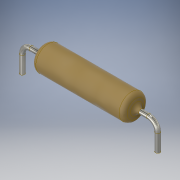
# Autodesk Inventor part: Resistor_TH-15mm
Saved by Autodesk Inventor 2018 (Build 220112000, 112)
## iProperties
Created: 2018-07-06
Part Number: Resistor_TH-15mm
Material: Copper
Document SubType Name: Modeling
Designer: Bradley
Density: 8.94 g/cm^3
Appearance: Textured - Dark Gold
Mass: 1.31337 g
Surface Area: 1.83215 cm^2
Volume: 0.14691 cm^3
Author: Bradley
Autodesk Inventor part; units mm, degrees
ref_plane "YZ Plane" through (0, 0, 0) normal (1, 0, 0) x (0, 1, 0)
ref_plane "XZ Plane" through (0, 0, 0) normal (0, 1, 0) x (-1, 0, 0)
ref_plane "XY Plane" through (0, 0, 0) normal (0, 0, 1) x (1, 0, 0)
sketch "Sketch1" plane through (0, 0, 0) normal (0, 0, 1) x (1, 0, 0)
  line L0 (-5.6474, 0) -> (5.6474, 0)
  line L1 (5.6474, 0) -> (5.6474, 0.254)
  arc A0 (5.155, 0.6672) -> (5.6474, 0.254) centre (5.6474, 0.754) ccw
  line L2 (5.155, 0.6672) -> (5.0995, 0.9818)
  arc A1 (5.0995, 0.9818) -> (4.6071, 1.395) centre (4.6071, 0.895) ccw
  line L3 (-5.6474, 0) -> (-5.6474, 0.254)
  arc A2 (-5.6474, 0.254) -> (-5.155, 0.6672) centre (-5.6474, 0.754) ccw
  line L4 (-5.155, 0.6672) -> (-5.0995, 0.9818)
  arc A3 (-4.6071, 1.395) -> (-5.0995, 0.9818) centre (-4.6071, 0.895) ccw
  line L5 (-4.6071, 1.395) -> (4.6071, 1.395)
  point P0 (0, 0)
  point P1 (0, 0)
  dimension "d0" = 2.79
  dimension "d1" = 0.508
  dimension "d2" = 10.31
  dimension "d3" = 0.5
  dimension "d6" = 0.5
  dimension "d7" = 80
  constraints: 12 end point, 10 point on circle, 6 tangent, 4 centre point, 2 equal length, 2 equal radius, 2 horizontal, 2 point on line, 1 coincident, 1 midpoint, 1 perpendicular, 1 vertical
  measures "d0" diameter of L5 L0
  measures "d1" diameter of L3.end L0
  measures "d2" distance of L2.start L4.start
  measures "d3" radius of A2
  measures "d6" radius of A3
  measures "d7" angle of L0 L4
revolve "Revolution1" add sketch "Sketch1" angle 360 about axis through (-5.6474, 0, 0) along (1, 0, 0)
sketch "Sketch2" plane through (0, 0, 0) normal (0, 0, 1) x (1, 0, 0)
  line L0 (-5.6474, -0.254) -> (-5.6474, 0.254) projected
  line L1 (5.6474, -0.254) -> (5.6474, 0.254) projected
  line L2 (-7.5, -2.895) -> (-7.5, -1)
  arc A0 (-6.5, 0) -> (-7.5, -1) centre (-6.5, -1) ccw
  line L3 (-6.5, 0) -> (6.5, 0)
  arc A1 (7.5, -1) -> (6.5, 0) centre (6.5, -1) ccw
  line L4 (7.5, -1) -> (7.5, -2.895)
  arc A2 (-5.0995, -0.9818) -> (-4.6071, -1.395) centre (-4.6071, -0.895) ccw projected
  point P0 (0, 0)
  point P1 (0, 0)
  point P2 (-4.6071, -1.395)
  dimension "d9" = 1
  dimension "d10" = 0.8526
  dimension "d11" = 15
  dimension "d12" = 2.895
  dimension "d13" = 1.5
  constraints: 6 end point, 5 point on circle, 4 tangent, 2 centre point, 1 coincident, 1 equal radius, 1 horizontal, 1 midpoint, 1 parallel, 1 perpendicular, 1 vertical, 1 vertical alignment
  measures "d9" radius of A0
  measures "d10" distance from line of L0 L3.start
  measures "d11" distance between parallel lines of L4 L2
  measures "d12" distance from line of L2.start L3
  measures "d13" vertical distance of L2.start point (-4.607, -1.395)
sketch "Sketch3" plane through (-5.6474, 0, 0) normal (-1, 0, 0) x (0, 0, 1)
  circle A0 centre (0, 0) radius 0.254 projected
sweep "Sweep1" add profiles "Sketch3" path "Sketch2" path curves L2 A0 L3 A1 L4
body "Solid1"
